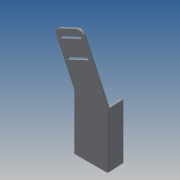
# Autodesk Inventor part: tow ribbon management
Saved by Autodesk Inventor 2013 (Build 170138000, 138)
## iProperties
Created: 2017-04-10
Part Number: tow ribbon management
Material: Generic
Document SubType Name: Modeling
Designer: employee
Density: 1 g/cm^3
Author: employee
Autodesk Inventor part; units mm, degrees
ref_plane "YZ Plane" through (0, 0, 0) normal (1, 0, 0) x (0, 1, 0)
ref_plane "XZ Plane" through (0, 0, 0) normal (0, 1, 0) x (-1, 0, 0)
ref_plane "XY Plane" through (0, 0, 0) normal (0, 0, 1) x (1, 0, 0)
sketch "Sketch1" plane through (0, 0, 0) normal (0, 0, 1) x (1, 0, 0)
  line L0 (-13, 0) -> (13, 0)
  line L1 (13, 0) -> (12.25, 13)
  line L2 (12.25, 13) -> (14.2533, 13)
  line L3 (15, -2) -> (-15, -2)
  line L4 (-14.2533, 13) -> (-12.25, 13)
  line L5 (-12.25, 13) -> (-13, 0)
  line L6 (-15, -2) -> (-15, 0.0576)
  line L7 (-15, 0.0576) -> (-14.2533, 13)
  line L8 (15, -2) -> (15, 0.0576)
  line L9 (15, 0.0576) -> (14.2533, 13)
  point P0 (0, 0)
  point P1 (0, 0)
  point P2 (0, -2)
  dimension "d0" = 24.5
  dimension "d2" = 2
  dimension "d4" = 26
  dimension "d5" = 13
  dimension "d27" = 2
  dimension "d28" = 2
  constraints: 20 end point, 6 parallel, 2 equal length, 2 midpoint, 1 coincident, 1 horizontal, 1 horizontal alignment, 1 perpendicular, 1 vertical alignment
  measures "d0" distance of L1.end L4.end
  measures "d2" distance between parallel lines of L0 L3
  measures "d4" distance of L0.start L0.end
  measures "d5" distance from line of L4.start L0
  measures "d27" distance between parallel lines of L7 L5
  measures "d28" distance from line of L6 L0.start
extrude "Extrusion1" add sketch "Sketch1" along normal blind 50
sketch "Sketch2" plane through (-15, -2, 0) normal (0, -1, 0) x (1, 0, 0)
  line L0 (0, 50) -> (30, 50) projected
  line L1 (0, 0) -> (0, 50) projected
  line L2 (15, 50) -> (-6.1309, 95.3154)
  line L3 (-18.4518, 89.5701) -> (6.19, 101.0607)
  line L4 (6.19, 101.0607) -> (27.3209, 55.7453)
  line L5 (27.3209, 55.7453) -> (2.6791, 44.2547)
  line L6 (2.6791, 44.2547) -> (-18.4518, 89.5701)
  line L7 (30, 50) -> (27.3209, 55.7453)
  point P0 (15, 0)
  dimension "d8" = 25
  dimension "d13" = 50
  constraints: 12 end point, 4 midpoint, 3 parallel, 2 perpendicular, 1 point on line
  measures "d8" angle of L2 L1
  measures "d13" distance between parallel lines of L5 L3
extrude "Extrusion2" add sketch "Sketch2" against normal up to surface (2 mm away)
sketch "Sketch3" plane through (-15, -2, 0) normal (0, -1, 0) x (1, 0, 0)
  line L0 (30, 0) -> (30, 50) projected
  line L1 (6.19, 101.0607) -> (-18.4518, 89.5701) projected
  line L2 (-18.4518, 89.5701) -> (0, 50) projected
  line L3 (-13.5341, 86.3464) -> (-12.6888, 84.5337)
  line L4 (-12.6888, 84.5337) -> (6.3436, 93.4087)
  line L5 (6.3436, 93.4087) -> (5.4984, 95.2213)
  line L6 (5.4984, 95.2213) -> (-13.5341, 86.3464)
  line L7 (-6.1309, 95.3154) -> (30, 17.8324) construction
  point P0 (30.2374, 50)
  point P1 (15, 0)
  point P2 (-4.0178, 90.7839)
  dimension "d17" = 21
  dimension "d19" = 5
  dimension "d20" = 2
  constraints: 10 end point, 3 parallel, 2 midpoint, 2 perpendicular, 1 point on line, 2 other
  measures "d17" distance of L5.end L3.start
  measures "d19" distance between parallel lines of L1 L6
  measures "d20" distance between parallel lines of L6 L4
extrude "Extrusion3" cut sketch "Sketch3" against normal through all
pattern_linear "Rectangular Pattern1" count 2 spacing 15 along (0.4226, 0, -0.9063) of "Extrusion3"
fillet "Fillet1" radius 5 2 edges at (-33.4518, -1, 89.5701) (-8.81, -1, 101.0607)
body "Solid1"
